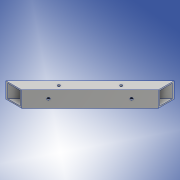
# Autodesk Inventor part: C002
Saved by Autodesk Inventor 2017 SP1 (Build 210196100, 196)
## iProperties
Created: 2017-06-13
Part Number: C002
Material: Aluminum 6061
Document SubType Name: Modeling
Designer: zallen
Density: 2.7 g/cm^3
Appearance: Aluminum - Flat
Mass: 30.515 g
Surface Area: 153.189 cm^2
Volume: 11.3018 cm^3
Author: zallen
Autodesk Inventor part; units mm, degrees
ref_plane "YZ Plane" through (0, 0, 0) normal (1, 0, 0) x (0, 1, 0)
ref_plane "XZ Plane" through (0, 0, 0) normal (0, 1, 0) x (-1, 0, 0)
sketch "Sketch1" plane through (0, 0, 0) normal (0, 0, 1) x (1, 0, 0)
  line L0 (0, 0) -> (100, 0) construction
  line L1 (100, 0) -> (100, 100) construction
  line L2 (100, 100) -> (0, 100) construction
  line L3 (0, 100) -> (0, 0) construction
  line L4 (0, 0) -> (100, 100)
  line L5 (0, 0) -> (19, 0)
  line L6 (100, 100) -> (100, 81)
  line L7 (19, 0) -> (100, 81)
  dimension "d1" = 100
  dimension "d2" = 100
  dimension "d3" = 19
  dimension "d4" = 19
  constraints: 16 end point, 2 parallel, 2 point on line, 1 horizontal, 1 perpendicular
  measures "d1" distance of L2.end L1.end
  measures "d2" distance of L1.end L0.end
  measures "d3" distance of L0.start L5.end
  measures "d4" distance of L1.end L6.end
extrude "Extrusion1" add sketch "Sketch1" along normal blind 19
ref_plane "Work Plane1" through (59.5, 40.5, 19) normal (-0.7071, -0.7071, 0) x (-0.7071, 0.7071, 0)
sketch "Sketch2" plane through (59.5, 40.5, 19) normal (-0.7071, -0.7071, 0) x (-0.7071, 0.7071, 0)
  line L0 (13.435, 19) -> (0, 19) projected
  line L1 (13.435, 19) -> (13.435, 0) projected
  line L2 (0, 0) -> (13.435, 0) projected
  line L3 (0, 19) -> (0, 0) projected
  line L4 (11.935, 1.5) -> (11.935, 17.5)
  line L5 (11.935, 17.5) -> (1.5, 17.5)
  line L6 (1.5, 17.5) -> (1.5, 1.5)
  line L7 (1.5, 1.5) -> (11.935, 1.5)
  point P0 (13.435, 19)
  dimension "d7" = 1.5
  constraints: 8 end point, 3 other
  measures "d7" distance between parallel lines of L2 L7
extrude "Extrusion2" cut sketch "Sketch2" along normal through all both and the other way through all contours L7 L6 L5 L4
sketch "Sketch4" plane through (0, 0, 19) normal (0, 0, 1) x (1, 0, 0)
  line L0 (36.3882, 26.4887) -> (73.5113, 63.6118) construction
  line L1 (54.9497, 45.0503) -> (50, 50) construction
  line L2 (100, 100) -> (0, 0) construction
  circle A0 centre (36.3882, 26.4887) radius 1.5
  circle A1 centre (73.5113, 63.6118) radius 1.5
  line L3 (19, 0) -> (100, 81) projected
  dimension "d22" = 52.5
  dimension "d24" = 7
  dimension "d25" = 3
  dimension "d26" = 3
  constraints: 4 end point, 2 centre point, 2 coincident, 2 midpoint, 2 perpendicular
  measures "d22" distance of L0.start L0.end
  measures "d24" distance of L1.start L1.end
  measures "d25" diameter of A0
  measures "d26" diameter of A1
extrude "Extrusion4" cut sketch "Sketch4" against normal through all
sketch "Sketch5" plane through (100, 81, 19) normal (0.7071, -0.7071, 0) x (-0.7071, -0.7071, 0)
  line L0 (92.2756, 9) -> (22.2756, 9) construction
  line L1 (0, 19) -> (114.5513, 19) projected
  circle A0 centre (92.2756, 9) radius 1.5
  circle A1 centre (22.2756, 9) radius 1.5
  point P0 (127.9863, 19)
  point P1 (57.2756, 19)
  point P2 (57.2756, 9)
  dimension "d29" = 70
  dimension "d30" = 10
  dimension "d31" = 3
  dimension "d32" = 3
  constraints: 2 centre point, 2 coincident, 2 end point, 2 midpoint, 1 horizontal, 1 vertical alignment
  measures "d29" distance of L0.start L0.end
  measures "d30" distance between parallel lines of L1 L0
  measures "d31" diameter of A0
  measures "d32" diameter of A1
extrude "Extrusion5" cut sketch "Sketch5" against normal through all
body "Solid1"
